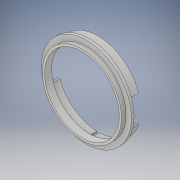
# Autodesk Inventor part: Teesiebhalter
Saved by Autodesk Inventor 2017 (Build 210142000, 142)
## iProperties
Part Number: Teesiebhalter
Material: Generisch
Document SubType Name: Modeling
Designer: OleSi
Density: 1 g/cm^3
Appearance: Vorgabe
Author: OleSi
Autodesk Inventor part; units mm, degrees
ref_plane "YZ Plane" through (0, 0, 0) normal (1, 0, 0) x (0, 1, 0)
ref_plane "XZ Plane" through (0, 0, 0) normal (0, 1, 0) x (-1, 0, 0)
ref_plane "XY Plane" through (0, 0, 0) normal (0, 0, 1) x (1, 0, 0)
sketch "Skizze1" plane through (0, 0, 0) normal (0, 1, 0) x (-1, 0, 0)
  circle A0 centre (0, 0) radius 45
  circle A1 centre (0, 0) radius 47.5
  dimension "d0" = 90
  dimension "d1" = 95
  constraints: 2 centre point, 2 coincident
  measures "d0" diameter of A0
  measures "d1" diameter of A1
extrude "Extrusion1" add sketch "Skizze1" along normal blind 10
sketch "Skizze2" plane through (0, 0, 0) normal (0, -1, 0) x (1, 0, 0)
  circle A0 centre (0, 0) radius 41.5
  circle A1 centre (0, 0) radius 50
  dimension "d4" = 83
  dimension "d5" = 100
  constraints: 2 centre point, 2 coincident
  measures "d4" diameter of A0
  measures "d5" diameter of A1
extrude "Extrusion2" add sketch "Skizze2" along normal blind 3
sketch "Skizze3" plane through (0, -3, 0) normal (0, -1, 0) x (1, 0, 0)
  circle A0 centre (0, 0) radius 41.5
  circle A1 centre (0, 0) radius 44
  dimension "d8" = 83
  dimension "d9" = 88
  constraints: 2 centre point, 2 coincident
  measures "d8" diameter of A0
  measures "d9" diameter of A1
extrude "Extrusion3" add sketch "Skizze3" along normal blind 5
sketch "Skizze4" plane through (0, 0, 0) normal (0, 1, 0) x (1, 0, 0)
  line L0 (-86, 0) -> (65, 0) construction
  line L1 (-86, 15) -> (65, 15)
  line L2 (-86, -15) -> (65, -15)
  line L3 (-86, 15) -> (-86, -15)
  line L4 (65, -15) -> (65, 15)
  point P0 (0, 0)
  dimension "d12" = 15
  dimension "d13" = 15
  constraints: 10 end point, 3 parallel, 1 horizontal, 1 point on line, 1 vertical
  measures "d12" distance between parallel lines of L0 L1
  measures "d13" distance between parallel lines of L0 L2
extrude "Extrusion4" cut sketch "Skizze4" along normal up to surface (10 mm away)
sketch "Skizze5" plane through (0, 10, 0) normal (0, 1, 0) x (1, 0, 0)
  line L0 (0, 0) -> (0, 69) construction
  line L1 (-1.5, 0) -> (-1.5, 46.3972)
  line L2 (1.5, 0) -> (1.5, 46.3972)
  line L3 (-1.5, 0) -> (1.5, 0)
  line L4 (-1.5, 46.3972) -> (1.5, 46.3972)
  dimension "d16" = 1.5
  constraints: 10 end point, 3 parallel, 1 horizontal
  measures "d16" distance between parallel lines of L0 L1
extrude "Extrusion5" cut sketch "Skizze5" against normal up to surface (10 mm away)
